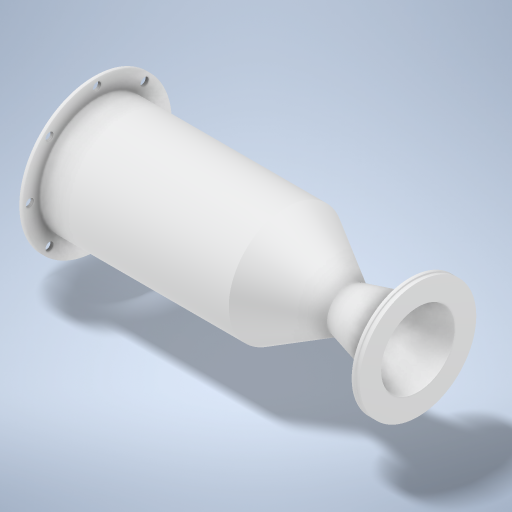
# Autodesk Inventor part: aluminium engine
Saved by Autodesk Inventor 2023 (Build 270158000, 158)
## iProperties
Created: 2022-09-15
Part Number: aluminium engine
Material: Aluminum 6061
Document SubType Name: Modeling
Designer: station
Density: 2.7 g/cm^3
Appearance: Aluminum - Flat
Author: station
Autodesk Inventor part; units mm, degrees
ref_plane "YZ Plane" through (0, 0, 0) normal (1, 0, 0) x (0, 1, 0)
ref_plane "XZ Plane" through (0, 0, 0) normal (0, 1, 0) x (-1, 0, 0)
ref_plane "XY Plane" through (0, 0, 0) normal (0, 0, 1) x (1, 0, 0)
sketch "Sketch2" plane through (0, 0, 0) normal (0, 0, 1) x (1, 0, 0)
  line L0 (0, 54.5) -> (192, 54.5)
  line L1 (254.7886, 18.124) -> (254.7886, 0) construction
  line L2 (192, 54.5) -> (254.7886, 18.124)
  line L3 (254.7886, 18.124) -> (325.1228, 36.97)
  line L4 (254.7886, 18.124) -> (254.7886, 43.3259) construction
  line L5 (0, 0) -> (254.7886, 0)
  line L6 (325.1228, 36.97) -> (325.1228, 0)
  line L7 (192, 54.5) -> (254.7886, 18.124)
  line L8 (325.1228, 0) -> (305.1228, 0)
  line L9 (-65.0246, 0) -> (390.1474, 0) projected
  line L10 (0, 57.5) -> (192, 57.5)
  line L11 (193.5039, 57.0958) -> (255.2149, 21.3441)
  line L12 (255.2149, 21.3441) -> (325.1228, 40.0758)
  line L13 (325.1228, 36.97) -> (325.1228, 40.0758)
  line L14 (0, 54.5) -> (0, 57.5)
  line L15 (193.5039, 57.0958) -> (192.8038, 57.5)
  line L16 (193.5039, 57.0958) -> (200.0085, 57.0958) construction
  line L17 (192, 57.5) -> (192.8038, 57.5)
  line L18 (325.1228, 40.0758) -> (325.1228, 57.5)
  line L19 (317.1228, 57.5) -> (317.1228, 37.9322)
  line L20 (325.1228, 0) -> (325.1228, 58.5)
  line L21 (317.1228, 58.5) -> (317.1228, 57.5)
  line L22 (317.1228, 58.5) -> (325.1228, 58.5)
  point P0 (254.7886, 31.9804)
  point P1 (325.1228, 59.5)
  point P2 (321.1228, 58.5)
  dimension "d2" = 18.124
  dimension "d9" = 54.5
  dimension "d43" = 192
  dimension "d76" = 20
  dimension "d141" = 3
  dimension "d142" = 3
  dimension "d143" = 3
  dimension "d144" = 150
  dimension "d159" = 8
  dimension "d199" = 58.5
  constraints: 44 end point, 5 vertical, 3 horizontal, 3 point on line, 2 parallel, 1 collinear, 1 midpoint, 1 perpendicular
  measures "d2" distance of L1.start L1.end
  measures "d9" distance from line of L5.start L0
  measures "d43" distance of L0.start L0.end
  measures "d76" distance of L6.end L8.end
  measures "d141" distance between parallel lines of L0 L10
  measures "d142" distance between parallel lines of L2 L11
  measures "d143" distance between parallel lines of L3 L12
  measures "d144" angle of L16 L15
  measures "d159" distance of L18.end L19.start
  measures "d199" distance from line of L8 point (321.123, 58.5)
revolve "Revolution1" add sketch "Sketch2" angle 360 about axis through (0, 0, 0) along (1, 0, 0) contours L14 L10 L17 L15 L11 L12 L13 L3 L2 L0
sketch "Sketch24" plane through (0, 0, 0) normal (-1, 0, 0) x (0, 0, 1)
  circle A0 centre (0, 0) radius 75
  circle A1 centre (0, 0) radius 21.3441 projected
  circle A2 centre (0, 0) radius 57.5
  dimension "d155" = 150
  dimension "d156" = 115
  constraints: 2 centre point, 2 coincident
  measures "d155" diameter of A0
  measures "d156" diameter of A2
extrude "Extrusion9" add sketch "Sketch24" against normal blind 3 contours A0
revolve "Revolution4" add sketch "Sketch2" angle 360 about axis through (-10, 0, 0) along (1, 0, 0) contours L12 L19 L21 L22 L20 L18
sketch "Sketch25" plane through (0, 0, 0) normal (0, 0, 1) x (1, 0, 0)
  line L0 (317.1228, -54.5) -> (317.1228, 54.5) projected
  line L1 (317.1228, 54.5) -> (320.1228, 54.5)
  line L2 (317.1228, 54.5) -> (325.1228, 54.5) projected
  line L3 (320.1228, 54.5) -> (320.1228, 53.5)
  line L4 (320.1228, 53.5) -> (322.1228, 53.5)
  line L5 (322.1228, 53.5) -> (322.1228, 54.5)
  line L6 (322.1228, 54.5) -> (320.7933, 54.5)
  line L7 (317.1228, -58.5) -> (317.1228, 58.5) projected
  line L8 (317.1228, 54.5) -> (317.1228, 58.5)
  line L9 (320.1189, 58.348) -> (320.0429, 56.8499)
  line L10 (317.1228, 58.5) -> (320.1228, 58.5)
  line L11 (317.1228, 58.5) -> (325.1228, 58.5) projected
  line L12 (320.1228, 58.5) -> (320.0506, 57.0017)
  point P0 (0, 0)
  dimension "d161" = 3
  dimension "d162" = 1
  dimension "d163" = 2
  dimension "d202" = 3
  constraints: 18 end point, 5 point on line, 3 perpendicular, 1 collinear
  measures "d161" distance of L0.end L1.end
  measures "d162" distance of L1.end L3.end
  measures "d163" distance of L3.end L4.end
  measures "d202" distance of L7.end L10.end
revolve "Revolution5" [suppressed]
sketch "Sketch26" plane through (0, 0, 0) normal (-1, 0, 0) x (0, 0, 1)
  circle A0 centre (0, 0) radius 18.124 projected
  circle A1 centre (0, 0) radius 67.5
  circle A2 centre (0, 67.5) radius 4
  circle A3 centre (-47.7297, 47.7297) radius 4
  circle A4 centre (-67.5, 0) radius 4
  circle A5 centre (-47.7297, -47.7297) radius 4
  circle A6 centre (0, -67.5) radius 4
  circle A7 centre (47.7297, -47.7297) radius 4
  circle A8 centre (67.5, 0) radius 4
  circle A9 centre (47.7297, 47.7297) radius 4
  point P0 (0, 0)
  dimension "d165" = 135
  dimension "d166" = 8
  dimension "d169" = 360
  constraints: 8 centre point, 1 coincident, 1 vertical alignment, 19 other
  measures "d166" diameter of A2
hole "Hole1" at (0, 67.5, 0) at (0, 47.7297, -47.7297) at (0, 0, -67.5) at (0, 47.7297, 47.7297) at (0, 0, 67.5) at (0, -47.7297, -47.7297) at (0, -67.5, 0) at (0, -47.7297, 47.7297) direction (1, 0, 0) diameter 8 end through all
thread "Thread19" size "M8x1.25" class "6H" standard "ANSI Metric M Profile" full length
thread "Thread20" size "M8x1.25" class "6H" standard "ANSI Metric M Profile" full length
thread "Thread21" size "M8x1.25" class "6H" standard "ANSI Metric M Profile" full length
thread "Thread22" size "M8x1.25" class "6H" standard "ANSI Metric M Profile" full length
thread "Thread23" size "M8x1.25" class "6H" standard "ANSI Metric M Profile" full length
thread "Thread24" size "M8x1.25" class "6H" standard "ANSI Metric M Profile" full length
thread "Thread25" size "M8x1.25" class "6H" standard "ANSI Metric M Profile" full length
thread "Thread26" size "M8x1.25" class "6H" standard "ANSI Metric M Profile" full length
thread "Thread27" size "M8x1.25" class "6H" standard "ANSI Metric M Profile" full length
sketch "Sketch27" plane through (0, 0, 0) normal (0, 0, 1) x (1, 0, 0)
  line L0 (317.1228, -58.5) -> (317.1228, 58.5) projected
  line L1 (317.1228, 58.5) -> (320.1228, 58.5)
  line L2 (317.1228, 58.5) -> (325.1228, 58.5) projected
  line L3 (320.1228, 58.5) -> (320.1228, 57)
  line L4 (320.1228, 57) -> (322.1228, 57)
  line L5 (322.1228, 57) -> (322.1228, 58.5)
  line L6 (-65.0246, 0) -> (390.1474, 0) projected
  point P0 (0, 0)
  dimension "d207" = 3
  dimension "d208" = 1.5
  dimension "d209" = 2
  constraints: 8 end point, 3 perpendicular, 2 point on line
  measures "d207" distance of L0.end L1.end
  measures "d208" distance of L1.end L3.end
  measures "d209" distance of L3.end L4.end
revolve "Revolution6" cut sketch "Sketch27" angle 360 about axis through (-10, 0, 0) along (1, 0, 0)
body "Solid1"
